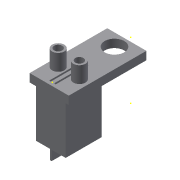
# Autodesk Inventor part: jtd_lid4_20160910
Saved by Autodesk Inventor 2016 (Build 200138000, 138)
## iProperties
Created: 2015-06-17
Part Number: jtd_lid4_20160910
Material: Generic
Document SubType Name: Modeling
Designer: Daniel
Density: 1 g/cm^3
Appearance: Default
Mass: 10.1656 g
Surface Area: 123.674 cm^2
Volume: 10.1656 cm^3
Author: Daniel
Autodesk Inventor part; units mm, degrees
ref_plane "YZ Plane" through (0, 0, 0) normal (1, 0, 0) x (0, 1, 0)
ref_plane "XZ Plane" through (0, 0, 0) normal (0, 1, 0) x (-1, 0, 0)
sketch "Sketch1" plane through (0, 0, 0) normal (0, 1, 0) x (-1, 0, 0)
  line L0 (12, 50) -> (-12, 50)
  line L1 (-12, 50) -> (-12, -50)
  line L2 (-12, -50) -> (12, -50)
  line L3 (12, -50) -> (12, 50)
  line L4 (12, 50) -> (-12, -50) construction
  line L5 (-12, 50) -> (12, -50) construction
  point P0 (0, 0)
  dimension "d0" = 24
  dimension "d1" = 100
  dimension "d135" = 50
  constraints: 12 end point, 2 midpoint, 2 parallel, 1 horizontal, 1 perpendicular
  measures "d0" distance of L1.end L2.end
  measures "d1" distance of L2.end L0.start
  measures "d135" distance from line of L2 point (0, 0)
extrude "Extrusion1" add sketch "Sketch1" along normal blind 5
sketch "Sketch3" plane through (0, 5, 0) normal (0, 1, 0) x (1, 0, 0)
  line L0 (-0.2475, -27) -> (0.2525, -27)
  line L1 (0.2525, -27) -> (0.2525, -49)
  line L2 (0.2525, -49) -> (-0.2475, -49)
  line L3 (-0.2475, -49) -> (-0.2475, -27)
  line L4 (12, -50) -> (12, 50) projected
  line L5 (-12, 50) -> (-12, -50) projected
  line L6 (-12, -50) -> (12, -50) projected
  point P0 (0, 0)
  dimension "d24" = 0.5
  dimension "d25" = 11.7475
  dimension "d26" = 22
  dimension "d97" = 11.7525
  dimension "d113" = 1
  constraints: 8 end point, 2 parallel, 1 horizontal, 1 perpendicular
  measures "d24" distance of L0.start L0.end
  measures "d25" distance between parallel lines of L4 L1
  measures "d26" distance of L0.end L1.end
  measures "d97" distance between parallel lines of L5 L3
  measures "d113" distance from line of L6 L1.end
extrude "Extrusion3" add sketch "Sketch3" along normal blind 30
sketch "Sketch4" plane through (0, 5, 0) normal (0, 1, 0) x (1, 0, 0)
  line L0 (-9.1, -27) -> (9.1, -27)
  line L1 (9.1, -27) -> (9.1, -28)
  line L2 (9.1, -28) -> (-9.1, -28)
  line L3 (-9.1, -28) -> (-9.1, -27)
  line L4 (12, -50) -> (12, 50) projected
  line L5 (-12, 50) -> (-12, -50) projected
  line L6 (-12, -50) -> (12, -50) projected
  point P0 (0, 0)
  dimension "d29" = 1
  dimension "d30" = 2.9
  dimension "d31" = 2.9
  dimension "d114" = 22
  constraints: 8 end point, 2 parallel, 1 horizontal, 1 perpendicular
  measures "d29" distance of L0.end L1.end
  measures "d30" distance between parallel lines of L4 L1
  measures "d31" distance between parallel lines of L5 L3
  measures "d114" distance between parallel lines of L6 L2
extrude "Extrusion4" add sketch "Sketch4" along normal blind 30
sketch "Sketch7" plane through (0, 5, 0) normal (0, 1, 0) x (1, 0, 0)
  line L0 (9.1, -27) -> (8.1, -27)
  line L1 (8.1, -27) -> (8.1, -49)
  line L2 (8.1, -49) -> (9.1, -49)
  line L3 (9.1, -49) -> (9.1, -27)
  line L4 (12, -50) -> (12, 50) projected
  point P0 (0, 0)
  dimension "d46" = 22
  dimension "d47" = 2.9
  dimension "d48" = 1
  constraints: 8 end point, 2 parallel, 1 horizontal, 1 perpendicular
  measures "d46" distance of L2.end L0.start
  measures "d47" distance between parallel lines of L4 L3
  measures "d48" distance of L1.end L2.end
extrude "Extrusion7" add sketch "Sketch7" along normal blind 30
sketch "Sketch8" plane through (0, 5, 0) normal (0, 1, 0) x (1, 0, 0)
  line L0 (-9.1, -28) -> (-8.1, -28)
  line L1 (-8.1, -28) -> (-8.1, -49)
  line L2 (-8.1, -49) -> (-9.1, -49)
  line L3 (-9.1, -49) -> (-9.1, -28)
  line L4 (-12, 50) -> (-12, -50) projected
  point P0 (0, 0)
  dimension "d51" = 21
  dimension "d52" = 2.9
  dimension "d53" = 1
  constraints: 8 end point, 2 parallel, 1 horizontal, 1 perpendicular
  measures "d51" distance of L2.end L0.start
  measures "d52" distance between parallel lines of L4 L3
  measures "d53" distance of L1.end L2.end
extrude "Extrusion8" add sketch "Sketch8" along normal blind 30
sketch "Sketch9" plane through (0, 5, 0) normal (0, 1, 0) x (1, 0, 0)
  line L0 (-8.3501, -48) -> (-0.2475, -48)
  line L1 (-0.2475, -48) -> (-0.2475, -49)
  line L2 (-0.2475, -49) -> (-8.3501, -49)
  line L3 (-8.3501, -49) -> (-8.3501, -48)
  line L4 (-0.2475, -49) -> (-0.2475, -27) projected
  line L5 (-12, -50) -> (12, -50) projected
  point P0 (0, 0)
  point P1 (-0.2475, -28)
  dimension "d56" = 8.1026
  dimension "d57" = 1
  dimension "d58" = 0
  dimension "d59" = 1
  constraints: 8 end point, 2 parallel, 1 horizontal, 1 perpendicular
  measures "d56" distance of L1.end L2.end
  measures "d57" distance of L0.end L1.end
  measures "d58" distance between parallel lines of L4 L1
  measures "d59" distance between parallel lines of L5 L2
extrude "Extrusion9" add sketch "Sketch9" along normal blind 30
sketch "Sketch10" plane through (0, 5, 0) normal (0, 1, 0) x (1, 0, 0)
  line L0 (0.2525, -48) -> (8.3551, -48)
  line L1 (8.3551, -48) -> (8.3551, -49)
  line L2 (8.3551, -49) -> (0.2525, -49)
  line L3 (0.2525, -49) -> (0.2525, -48)
  line L4 (-12, -50) -> (12, -50) projected
  line L5 (0.2525, -27) -> (0.2525, -49) projected
  point P0 (0, 0)
  point P1 (0.2525, -28)
  dimension "d62" = 8.1026
  dimension "d63" = 1
  dimension "d64" = 1
  dimension "d65" = 0
  constraints: 8 end point, 2 parallel, 1 horizontal, 1 perpendicular
  measures "d62" distance of L0.start L0.end
  measures "d63" distance between parallel lines of L4 L2
  measures "d64" distance of L2.end L0.start
  measures "d65" distance between parallel lines of L5 L3
extrude "Extrusion10" add sketch "Sketch10" along normal blind 30
sketch "Sketch11" plane through (0, 5, 0) normal (0, 1, 0) x (1, 0, 0)
  point P0 (0, 0)
sketch "Sketch12" plane through (0, 0, 0) normal (0, -1, 0) x (1, 0, 0)
  circle A0 centre (4.5, 43) radius 3.25
  line L0 (12, 50) -> (12, -50) projected
  circle A1 centre (-4.5, 43) radius 3.25
  line L1 (-12, -50) -> (-12, 50) projected
  line L2 (-12, 50) -> (12, 50) projected
  point P0 (0, 0)
  dimension "d69" = 6.5
  dimension "d70" = 7.5
  dimension "d72" = 6.5
  dimension "d73" = 7.5
  dimension "d74" = 7
  dimension "d75" = 7
  constraints: 2 centre point
  measures "d69" diameter of A0
  measures "d70" distance from line of L0 A0.centre
  measures "d72" diameter of A1
  measures "d73" distance from line of L1 A1.centre
  measures "d74" distance from line of L2 A0.centre
  measures "d75" distance from line of L2 A1.centre
extrude "Extrusion11" add sketch "Sketch12" along normal blind 20
sketch "Sketch15" plane through (4.5, -20, 43) normal (0, -1, 0) x (1, 0, 0)
  point P0 (-4.5, -43)
extrude "Extrusion12" [suppressed]
sketch "Sketch16" plane through (-4.5, -20, 43) normal (0, -1, 0) x (1, 0, 0)
  point P0 (4.5, -43)
extrude "Extrusion13" [suppressed]
ref_plane "Work Plane1" through (-12, 0, -50) normal (0, -1, 0) x (1, 0, 0)
split body "Split1" result two bodies by plane through (-12, 0, -50) normal (0, -1, 0) first body at (7.2144, -13.3333, 42.5589) (-1.7856, -13.3333, 42.5589)
split "Split2" plane through (-12, 0, -50) removes the side toward (0, -1, 0)
sketch "Sketch20" plane through (0, 0, 0) normal (0, -1, 0) x (1, 0, 0)
  line L0 (-1, 28) -> (-2, 28)
  line L1 (-2, 28) -> (-2, 48)
  line L2 (-2, 48) -> (-1, 48)
  line L3 (-1, 48) -> (-1, 28)
  line L4 (1, 28) -> (2, 28)
  line L5 (2, 28) -> (2, 48)
  line L6 (2, 48) -> (1, 48)
  line L7 (1, 48) -> (1, 28)
  line L8 (-12, -50) -> (-12, 50) projected
  line L9 (12, 50) -> (12, -50) projected
  line L10 (-12, 50) -> (12, 50) projected
  point P0 (0, 0)
  dimension "d84" = 11
  dimension "d85" = 11
  dimension "d86" = 1
  dimension "d87" = 1
  dimension "d88" = 20
  dimension "d89" = 2
  constraints: 16 end point, 4 parallel, 2 horizontal, 2 perpendicular, 2 point on line
  measures "d84" distance between parallel lines of L8 L3
  measures "d85" distance between parallel lines of L9 L7
  measures "d86" distance of L0.start L0.end
  measures "d87" distance of L4.start L4.end
  measures "d88" distance of L0.end L1.end
  measures "d89" distance from line of L10 L6.end
extrude "Extrusion14" cut sketch "Sketch20" against normal blind 25.4 bodies 3
sketch "Sketch25" plane through (0, 0, 0) normal (0, -1, 0) x (1, 0, 0)
  circle A0 centre (0, 10) radius 6
  line L0 (12, -50) -> (-12, -50) projected
  point P0 (0, 0)
  dimension "d109" = 12
  dimension "d110" = 60
  constraints: 1 centre point
  measures "d109" diameter of A0
  measures "d110" distance from line of L0 A0.centre
extrude "Extrusion18" cut sketch "Sketch25" against normal blind 25.4 bodies 3
sketch "Sketch26" plane through (0, 5, 0) normal (0, 1, 0) x (1, 0, 0)
  point P0 (0, 0)
sketch "Sketch27" plane through (-1, 0, 48) normal (0, 0, -1) x (-1, 0, 0)
  point P0 (-1, 0)
sketch "Sketch28" plane through (0, 5, 0) normal (0, 1, 0) x (1, 0, 0)
  point P0 (0, 0)
sketch "Sketch29" plane through (0, 0, 0) normal (0, -1, 0) x (1, 0, 0)
  circle A0 centre (-6.5, 38) radius 1.5
  circle A1 centre (6.5, 38) radius 1.5
  line L0 (-12, 50) -> (12, 50) projected
  line L1 (-12, -50) -> (-12, 50) projected
  line L2 (12, 50) -> (12, -50) projected
  point P0 (0, 0)
  dimension "d121" = 3
  dimension "d122" = 3
  dimension "d123" = 12
  dimension "d124" = 12
  dimension "d125" = 5.5
  dimension "d126" = 5.5
  constraints: 2 centre point
  measures "d121" diameter of A0
  measures "d122" diameter of A1
  measures "d123" distance from line of L0 A0.centre
  measures "d124" distance from line of L0 A1.centre
  measures "d125" distance from line of L1 A0.centre
  measures "d126" distance from line of L2 A1.centre
extrude "Extrusion19" cut sketch "Sketch29" against normal blind 25.4 bodies 3
sketch "Sketch30" plane through (0, 35, 0) normal (0, 1, 0) x (1, 0, 0)
  point P0 (0, 0)
sketch "Sketch31" plane through (0, 5, 0) normal (0, 1, 0) x (1, 0, 0)
  line L0 (-1, -28) -> (1, -28)
  line L1 (1, -28) -> (1, -48)
  line L2 (1, -48) -> (-1, -48)
  line L3 (-1, -48) -> (-1, -28)
  line L4 (-0.2475, -28) -> (-1, -28) projected
  line L5 (-1, -28) -> (-1, -48) projected
  line L6 (1, -48) -> (1, -28) projected
  line L7 (0.2525, -48) -> (1, -48) projected
  point P0 (0, 0)
  dimension "d129" = 0
  dimension "d130" = 0
  dimension "d131" = 0
  dimension "d132" = 0
  constraints: 8 end point, 2 parallel, 1 horizontal, 1 perpendicular
  measures "d129" distance between parallel lines of L4 L0
  measures "d130" distance between parallel lines of L5 L3
  measures "d131" distance between parallel lines of L6 L1
  measures "d132" distance between parallel lines of L7 L2
extrude "Extrusion20" add sketch "Sketch31" along normal blind 30 bodies 3
sketch "Sketch32" plane through (0, 0, 0) normal (0, -1, 0) x (1, 0, 0)
  point P0 (0, 0)
sketch "Sketch33" plane through (0, 0, 0) normal (0, -1, 0) x (1, 0, 0)
  point P0 (0, 0)
sketch "Sketch34" plane through (0, 0, 0) normal (0, -1, 0) x (1, 0, 0)
  point P0 (0, 0)
sketch "Sketch35" plane through (0, 5, 0) normal (0, 1, 0) x (1, 0, 0)
  point P0 (0, 0)
sketch "Sketch36" plane through (0, 5, 0) normal (0, 1, 0) x (1, 0, 0)
  point P0 (0, 0)
sketch "Sketch37" plane through (0, 5, 0) normal (0, 1, 0) x (1, 0, 0)
  point P0 (0, 0)
sketch "Sketch38" plane through (0, 5, 0) normal (0, 1, 0) x (1, 0, 0)
  point P0 (0, 0)
sketch "Sketch39" plane through (0, 5, 0) normal (0, 1, 0) x (1, 0, 0)
  point P0 (0, 0)
sketch "Sketch40" plane through (0, 5, 0) normal (0, 1, 0) x (1, 0, 0)
  line L0 (2, -28) -> (3, -28)
  line L1 (3, -28) -> (3, -48)
  line L2 (3, -48) -> (2, -48)
  line L3 (2, -48) -> (2, -28)
  line L4 (2, -48) -> (8.1, -48) projected
  line L5 (8.1, -28) -> (2, -28) projected
  point P0 (0, 0)
  dimension "d136" = 0
  dimension "d137" = 0
  dimension "d138" = 1
  dimension "d139" = 0
  constraints: 8 end point, 2 parallel, 1 horizontal, 1 perpendicular
  measures "d136" distance from line of L4 L1.end
  measures "d137" distance between parallel lines of L5 L0
  measures "d138" distance of L0.start L0.end
  measures "d139" distance of L5.end L0.start
extrude "Extrusion21" add sketch "Sketch40" along normal blind 30 bodies 3
sketch "Sketch41" plane through (0, 5, 0) normal (0, 1, 0) x (1, 0, 0)
  line L0 (-2, -28) -> (-3, -28)
  line L1 (-3, -28) -> (-3, -48)
  line L2 (-3, -48) -> (-2, -48)
  line L3 (-2, -48) -> (-2, -28)
  line L4 (-2, -28) -> (-8.1, -28) projected
  line L5 (-2, -48) -> (-2, -28) projected
  line L6 (-8.1, -48) -> (-2, -48) projected
  point P0 (0, 0)
  dimension "d142" = 0
  dimension "d143" = 0
  dimension "d144" = 0
  dimension "d145" = 1
  constraints: 8 end point, 2 parallel, 1 horizontal, 1 perpendicular
  measures "d142" distance between parallel lines of L4 L0
  measures "d143" distance between parallel lines of L5 L3
  measures "d144" distance between parallel lines of L6 L2
  measures "d145" distance of L1.end L2.end
extrude "Extrusion22" add sketch "Sketch41" along normal blind 30 bodies 3
sketch "Sketch42" plane through (0, 35, 0) normal (0, 1, 0) x (1, 0, 0)
  point P0 (0, 0)
sketch "Sketch43" plane through (0, 35, 0) normal (0, 1, 0) x (1, 0, 0)
  line L0 (9.1, -27) -> (-9.1, -27) projected
  line L1 (-9.1, -49) -> (9.1, -49) projected
  line L2 (-0.5, -27) -> (0.5, -27)
  line L3 (0.5, -27) -> (0.5, -49)
  line L4 (0.5, -49) -> (-0.5, -49)
  line L5 (-0.5, -49) -> (-0.5, -27)
  line L6 (1, -48) -> (1, -28) projected
  point P0 (0, 0)
  dimension "d148" = 1
  dimension "d149" = 0.5
  constraints: 8 end point, 2 parallel, 2 point on line, 1 horizontal, 1 perpendicular
  measures "d148" distance between parallel lines of L3 L5
  measures "d149" distance between parallel lines of L3 L6
extrude "baffle" add sketch "Sketch43" along normal blind 6 bodies 3
sketch "Sketch45" plane through (0, 0, 0) normal (0, -1, 0) x (1, 0, 0)
  circle A0 centre (-6.5, 38) radius 2.5
  circle A1 centre (-6.5, 38) radius 1.5 projected
  circle A2 centre (-6.5, 38) radius 3.7
  line L0 (-12, 50) -> (12, 50) projected
  line L1 (0, 50) -> (0, 16)
  circle A3 centre (0, 10) radius 6 projected
  circle A4 centre (6.5, 38) radius 2.5
  circle A5 centre (6.5, 38) radius 3.7
  point P0 (0, 0)
  dimension "d155" = 5
  dimension "d156" = 1.2
  constraints: 4 centre point, 2 end point, 2 symmetric about line, 1 coincident, 1 concentric, 1 midpoint, 1 perpendicular, 1 vertical, 1 vertical alignment, 3 other
  measures "d155" diameter of A0
  measures "d156" radial gap between concentric circles of A2 A0
extrude "Extrusion25" add sketch "Sketch45" along normal blind 10 contours A2 | A5 bodies 3
sketch "Sketch46" plane through (0, 5, 0) normal (0, 1, 0) x (1, 0, 0)
  line L0 (12, 50) -> (-12, 50) projected
  line L1 (12, -50) -> (12, 50) projected
  line L2 (-12, 50) -> (12, 50)
  line L3 (12, 50) -> (12, -2.4141)
  line L4 (12, -2.4141) -> (-12, -2.4141)
  line L5 (-12, -2.4141) -> (-12, 50)
  point P0 (0, 0)
  constraints: 8 end point, 2 parallel, 1 horizontal, 1 perpendicular, 1 point on line
extrude "Extrusion26" cut sketch "Sketch46" against normal through all bodies 3
body "Solid2"
body "Solid3"
